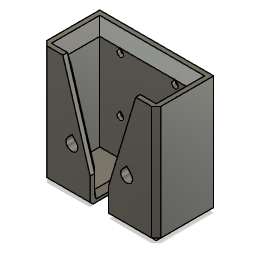
CNC_handrad_holder (Autodesk Fusion 360 design; units mm, degrees)
Autodesk Fusion 360 part; units mm, degrees
note: some values were not read from the file. Chosen so that the rebuilt part matches the saved one: which face or edge a step refers to; which pieces of a blend or face edit are solid. Set by a fixed rule: which sketch regions a step uses.
sketch "Sketch1" plane through (0, 0, 0) normal (0, 0, 1) x (1, 0, 0)
  line L0 (30, 30) -> (-30, 30) construction
  line L1 (-30, 30) -> (-30, -30) construction
  line L2 (-30, -30) -> (30, -30) construction
  line L3 (30, -30) -> (30, 30) construction
  line L4 (30, 30) -> (-30, -30) construction
  line L5 (-30, 30) -> (30, -30) construction
  circle A0 centre (-30, 30) radius 2.5
  circle A1 centre (30, 30) radius 2.5
  circle A2 centre (-30, -30) radius 2.5
  circle A3 centre (30, -30) radius 2.5
  line L6 (52.5, 50) -> (-52.5, 50)
  line L7 (-52.5, 50) -> (-52.5, -50)
  line L8 (-52.5, -50) -> (52.5, -50)
  line L9 (52.5, -50) -> (52.5, 50)
  line L10 (52.5, 50) -> (-52.5, -50) construction
  line L11 (-52.5, 50) -> (52.5, -50) construction
  line L12 (52.5, -50) -> (62.5, -50)
  line L13 (62.5, -50) -> (62.5, 50)
  line L14 (62.5, 50) -> (52.5, 50)
  line L15 (52.5, 50) -> (52.5, -50)
  line L16 (-52.5, -50) -> (-62.5, -50)
  line L17 (-62.5, -50) -> (-62.5, 50)
  line L18 (-62.5, 50) -> (-52.5, 50)
  line L19 (-52.5, 50) -> (-52.5, -50)
  line L20 (-62.5, -50) -> (62.5, -50)
  line L21 (62.5, -50) -> (62.5, -60)
  line L22 (62.5, -60) -> (-62.5, -60)
  line L23 (-62.5, -60) -> (-62.5, -50)
  line L24 (0, -60) -> (0, 50)
  line L25 (10, -60) -> (-10, -60)
  line L26 (-10, -60) -> (-10, -50)
  line L27 (-10, -50) -> (10, -50)
  line L28 (10, -50) -> (10, -60)
  line L29 (10, -60) -> (-10, -50) construction
  line L30 (-10, -60) -> (10, -50) construction
  line L31 (31.8432, -28.311) -> (30, -26.2995)
  line L32 (30, -26.2995) -> (28.1568, -28.311)
  line L33 (-28.1568, -28.311) -> (-30, -26.2995)
  line L34 (-30, -26.2995) -> (-31.8432, -28.311)
  line L35 (31.8432, 31.689) -> (30, 33.7005)
  line L36 (30, 33.7005) -> (28.1568, 31.689)
  line L37 (-28.1568, 31.689) -> (-30, 33.7005)
  line L38 (-30, 33.7005) -> (-31.8432, 31.689)
  circle A4 centre (-30, 30) radius 3.5
  circle A5 centre (30, 30) radius 3.5
  circle A6 centre (-30, -30) radius 3.5
  circle A7 centre (30, -30) radius 3.5
  line L39 (-32.5805, 32.3646) -> (-30, 35.1807)
  line L40 (-30, 35.1807) -> (-27.4195, 32.3646)
  line L41 (30, 35.1807) -> (32.5805, 32.3646)
  line L42 (27.4195, 32.3646) -> (30, 35.1807)
  line L43 (-30, -24.8193) -> (-27.4195, -27.6354)
  line L44 (-32.5805, -27.6354) -> (-30, -24.8193)
  line L45 (30, -24.8193) -> (32.5805, -27.6354)
  line L46 (27.4195, -27.6354) -> (30, -24.8193)
  point P0 (0, -55)
  dimension "d1" = 60
  dimension "d2" = 60
  dimension "d3" = 5
  dimension "d6" = 60
  dimension "d7" = -60
  dimension "d8" = 105
  dimension "d9" = 100
  dimension "d12" = 10
  dimension "d13" = 100
  dimension "d14" = 10
  dimension "d15" = 100
  dimension "d16" = 125
  dimension "d17" = 10
  dimension "d18" = 20
  dimension "d19" = 10
  dimension "d20" = 10
  dimension "d41" = 85
  dimension "d44" = -60
  dimension "d45" = 60
  dimension "d46" = 7
  dimension "d50" = 85
  constraint horizontal L0
  constraint perpendicular L0 L1
  constraint parallel L0 L2
  constraint parallel L1 L3
  constraint coincident L4 origin
  constraint coincident L5 origin
  constraint coincident L0.end L1.start
  constraint horizontal L6
  constraint perpendicular L6 L7
  constraint parallel L6 L8
  constraint parallel L7 L9
  constraint coincident L10 origin
  constraint coincident L11 origin
  constraint horizontal L12
  constraint vertical L13
  constraint horizontal L14
  constraint vertical L15
  constraint horizontal L16
  constraint vertical L17
  constraint horizontal L18
  constraint vertical L19
  constraint horizontal L20
  constraint vertical L21
  constraint horizontal L22
  constraint vertical L23
  constraint midpoint L22 L24.start
  constraint midpoint L6 L24.end
  constraint horizontal L25
  constraint perpendicular L25 L26
  constraint parallel L25 L27
  constraint parallel L26 L28
  constraint coincident L29 P0
  constraint coincident L30 P0
  constraint collinear L20 L27
  constraint coincident A3 L31.start
  constraint coincident L3 L31.end
  constraint tangent A3 L31
  constraint coincident A3 L32.end
  constraint tangent A3 L32
  constraint concentric A0 A4
  constraint coincident A4 L39.start
  constraint coincident A4 L40.end
  constraint tangent A4 L40
  constraint parallel L37 L40
  constraint tangent A4 L39
  measures "d1" distance of L1.end L2.end
  measures "d2" distance of L0.end L1.end
  measures "d3" diameter of A0
  measures "d8" distance of L7.end L8.end
  measures "d9" distance of L6.end L7.end
  measures "d12" distance of L8.end L12.end
  measures "d13" distance of L8.end L6.start
  measures "d14" distance of L7.end L16.end
  measures "d15" distance of L7.end L6.end
  measures "d16" distance of L16.end L12.end
  measures "d17" distance of L16.end L22.end
  measures "d18" distance of L26.end L27.end
  measures "d19" distance of L25.end L26.end
  measures "d20" distance of L24 L26
  measures "d41" angle of L31 L32
  measures "d46" diameter of A4
  measures "d50" angle of L39 L40
extrude "Extrude1" add sketch "Sketch1" along normal blind 10 contours A0 L37 L38 A4 | L37 L38 A4 L39 L40 | A1 L35 L36 A5 | L35 L36 A5 L41 L42 | A2 L33 L34 A6 | L33 L34 A6 L43 L44 | A3 L31 L32 A7 | L31 L32 A7 L45 L46 | L6 L8 L9 L15 L20 L24 L27 | L6 L7 L8 L19 L20 L24 L27 picked at (-30.8623, 26.9615) picked at (29.1377, 26.9615) picked at (-33.0959, -29.3746) picked at (32.7051, -31.6305) makes body 1
extrude "Extrude2" add sketch "Sketch1" along normal blind 53 contours L9 L12 L13 L14 L15 L20 | L8 L12 L20 L21 L22 L28 | L7 L16 L17 L18 L19 L20 | L8 L16 L20 L22 L23 L26 bodies 1
extrude "Extrude3" add sketch "Sketch1" along normal blind 10 from surface at 53 contours A0 L37 L38 A4 | A0 L37 L38 A4 | L37 L38 A4 | L37 L38 A4 L39 L40 | A1 L35 L36 A5 | A1 L35 L36 A5 | L35 L36 A5 | L35 L36 A5 L41 L42 | A2 L33 L34 A6 | A2 L33 L34 A6 | L33 L34 A6 | L33 L34 A6 L43 L44 | A3 L31 L32 A7 | A3 L31 L32 A7 | L31 L32 A7 | L31 L32 A7 L45 L46 | L6 L8 L9 L15 L20 L24 L27 | L9 L12 L13 L14 L15 L20 | L6 L7 L8 L19 L20 L24 L27 | L8 L12 L20 L21 L22 L28 | L7 L16 L17 L18 L19 L20 | L8 L16 L20 L22 L23 L26 bodies 1
extrude "Extrude4" cut 1 faces at (-3.3333, -50, 56.3333) along direction (0, 1, 0) blind 110 on bodies 1 bodies 1
chamfer "Chamfer1" distance 30 distance2 100 2 edges at (10, 50, 58) (-10, 50, 58) measured on face at (17.5, 50, 3.3333) measured on face at (17.5, 50, 3.3333) on bodies 1
chamfer "Chamfer2" distance 5 angle 45 4 edges at (10, -50, 31.5) (-10, -50, 31.5) (25, 0, 53) (-25, 0, 53) on bodies 1
extrude "Extrude5" add 1 faces at (-3.3333, -50, 3.3333) along direction (0, -1, 0) blind 10 on bodies 1 bodies 1
move_face "OffsetFaces1" offset -2 2 faces at (-27.5031, -30.1246, 59.6667) (32.4969, -30.1246, 59.6667) on bodies 1
chamfer "Chamfer3" distance 15 distance2 5 5 edges at (0, 50, 10) (-52.5, 50, 31.5) (52.5, 50, 31.5) (48.8601, 50, 53) (-48.8601, 50, 53) measured on face at (9.3904, -8.1012, 10) measured on face at (-52.5, 16.6667, 24.3333) measured on face at (17.5, 50, 3.3333) measured on face at (46.3515, -9.3492, 53) measured on face at (-46.3515, -9.3492, 53) on bodies 1
sketch "Sketch2" plane through (0, 0, 63) normal (0, 0, 1) x (1, 0, 0)
  line L0 (40, 50) -> (10, -50)
  line L1 (10, -50) -> (10, -60)
  line L2 (10, -60) -> (62.5, -60)
  line L3 (62.5, -60) -> (62.5, 50)
  line L4 (62.5, 50) -> (40, 50)
  circle A0 centre (30, -30) radius 4.5
  line L5 (30, -30) -> (30, -19.9992) construction
  line L6 (0, -61.23) -> (0, 33.77)
  circle A1 centre (30, -30) radius 6.5
  line L7 (25.2077, -25.6087) -> (30, -20.3788)
  line L8 (30, -20.3788) -> (34.7923, -25.6087)
  circle A2 centre (-30, -30) radius 6.5
  line L9 (-25.2077, -25.6087) -> (-30, -20.3788)
  line L10 (-30, -20.3788) -> (-34.7923, -25.6087)
  dimension "d38" = 13
  dimension "d51" = 85
  dimension "d52" = 60
  constraint coincident A0.centre L5.start
  constraint vertical L5
  constraint parallel L1 L6
  constraint concentric A0 A1
  constraint coincident A1 L7.start
  constraint coincident A1 L8.end
  constraint tangent A1 L7
  constraint tangent A1 L8
  constraint coincident L5 L7.end
  constraint symmetric L6 A1 A2
  constraint symmetric L6 L7.start L9.start
  constraint symmetric L6 L7.end L9.end
  constraint symmetric L6 L8.end L10.end
  measures "d38" diameter of A1
  measures "d51" angle of L7 L8
extrude "Extrude7" cut sketch "Sketch1" against normal blind 4 from surface at 10 contours A0 L37 L38 A4 | A0 L37 L38 A4 | L37 L38 A4 L39 L40 | A1 L35 L36 A5 | A1 L35 L36 A5 | L35 L36 A5 L41 L42 | A2 L33 L34 A6 | A2 L33 L34 A6 | L33 L34 A6 L43 L44 | A3 L31 L32 A7 | A3 L31 L32 A7 | L31 L32 A7 L45 L46 bodies 1
extrude "Extrude8" cut sketch "Sketch2" against normal blind 10 contours A1 | A1 L7 L8 | A2 | A2 L9 L10 bodies 1
ref_plane "WorkPlane1" through (0, -50, 31.5) normal (0, -1, 0) x (1, 0, 0)
split "Split1" by plane through (0, -50, 31.5) normal (0, -1, 0) bodies 1 makes body 2 at (-45, -60, 24.3333)
move_body "Move1" bodies 2 to x (1, 0, 0) y (0, 1, 0) z (0, 0, 1) at (0, -20, 0)
extrude "Extrude9" add 1 faces at (5, -50, 3.3333) along direction (0, -1, 0) blind 20 on bodies 1 bodies 1 2
chamfer "Chamfer4" distance 5 angle 45 6 edges at (-62.5, -80, 31.5) (-62.5, -15, 63) (-36.25, -80, 63) (62.5, -80, 31.5) (62.5, -15, 63) (36.25, -80, 63) on bodies 1
chamfer "Chamfer5" distance 2 angle 45 2 edges at (10, -80, 34) (-10, -80, 34) on bodies 1
